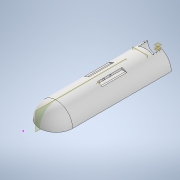
# Autodesk Inventor part: Корпус1
Saved by Autodesk Inventor 2022.1 (Build 261234000, 234)
## iProperties
Created: 2021-12-25
Part Number: Корпус1
Material: Типовые
Document SubType Name: Modeling
Designer: Grigori
Density: 1 g/cm^3
Appearance: По умолчанию
Author: Grigori
Autodesk Inventor part; units mm, degrees
ref_plane "YZ Plane" through (0, 0, 0) normal (1, 0, 0) x (0, 1, 0)
ref_plane "XZ Plane" through (0, 0, 0) normal (0, 1, 0) x (-1, 0, 0)
ref_plane "XY Plane" through (0, 0, 0) normal (0, 0, 1) x (1, 0, 0)
sketch "Эскиз1" plane through (0, 0, 0) normal (1, 0, 0) x (0, 1, 0)
  line L0 (100, -600) -> (0, -600)
  line L1 (0, -200) -> (0, -600)
  line L2 (0, -200) -> (0, -100)
  line L3 (100, -600) -> (100, -200)
  line L4 (100, -600) -> (500, -600) construction
  arc A0 (100, -200) -> (0, -100) centre (0, -200) ccw
  point P0 (0, 0)
  dimension "d0" = 100
  dimension "d4" = 100
  dimension "d42" = 400
  dimension "d43" = 90
  constraints: 10 end point, 3 vertical, 2 point on circle, 1 centre point, 1 coincident, 1 horizontal, 1 perpendicular
  measures "d0" distance of L0.start L0.end
  measures "d4" distance of L1.start L2.end
  measures "d42" distance of L3.end L0.start
  measures "d43" angle of L4 L3
extrude "Выдавливание1" add sketch "Эскиз1" along normal mid plane 500
sketch "Эскиз2" plane through (250, 100, -600) normal (0, 0, -1) x (-1, 0, 0)
  line L0 (500, -100) -> (0, -100) projected
  line L1 (-15.1415, -100) -> (-15.1415, 76.1146)
  line L2 (-15.1415, 76.1146) -> (561.5466, 76.1146)
  line L3 (561.5466, 76.1146) -> (561.5466, -100)
  line L4 (-15.1415, -100) -> (100, -100)
  line L5 (400, -100) -> (561.5466, -100)
  arc A0 (350, -100) -> (150, -100) centre (250, -100) ccw
  line L6 (100, -100) -> (150, -100)
  line L7 (350, -100) -> (400, -100)
  point P0 (150, -100)
  dimension "d44" = 200
  constraints: 14 end point, 2 collinear, 2 horizontal, 2 perpendicular, 2 point on circle, 1 centre point, 1 point on line, 1 vertical
  measures "d44" diameter of A0
extrude "Выдавливание5" cut sketch "Эскиз2" against normal through all contours L0 A0 L4 L1 L2 L3 L5
ref_plane "РабПлоскость6" through (0, 0, -600) normal (-1, 0, 0) x (0, -1, 0)
sketch "Эскиз9" plane through (0, 0, -600) normal (-1, 0, 0) x (0, -1, 0)
  arc A0 (0, 500) -> (-100, 400) centre (0, 400) ccw
  arc A1 (0, 591.5896) -> (-191.5896, 400) centre (0, 400) ccw
  line L0 (0, 400) -> (-247.1417, 400)
  line L1 (0, 400) -> (0, 629.865)
  line L2 (0, 500) -> (0, 0) projected
  point P0 (0, 600)
  constraints: 5 end point, 4 point on circle, 3 point on line, 2 centre point, 1 coincident, 1 collinear, 1 horizontal
revolve "Вращение3" cut sketch "Эскиз9" angle 360 about axis through (0, 0, -200) along (0, 0, 1) contours A0 L0 A1 L1
shell "Оболочка2" thickness 5 removed faces 1 at (33.3333, 0, -466.6667)
sketch "Эскиз11" plane through (-100, 0, -600) normal (0, -1, 0) x (1, 0, 0)
  line L0 (195, 400) -> (195, 5) projected
  line L1 (195, 5) -> (175, 5)
  line L2 (175, 5) -> (175, 25)
  line L3 (175, 25) -> (195, 25)
  line L4 (195, 25) -> (195, 5)
  line L5 (195, 5) -> (5, 5) projected
  line L6 (5, 5) -> (25, 5)
  line L7 (25, 5) -> (25, 25)
  line L8 (25, 25) -> (5, 25)
  line L9 (5, 25) -> (5, 5)
  line L10 (175, 385) -> (195, 385)
  line L11 (195, 385) -> (195, 365)
  line L12 (195, 365) -> (175, 365)
  line L13 (175, 365) -> (175, 385)
  line L14 (25, 385) -> (5, 385)
  line L15 (5, 385) -> (5, 365)
  line L16 (5, 365) -> (25, 365)
  line L17 (25, 365) -> (25, 385)
  point P0 (100, 600)
  dimension "d50" = 20
  dimension "d51" = 20
  dimension "d52" = 20
  dimension "d53" = 20
  dimension "d54" = 360
  dimension "d55" = 360
  dimension "d56" = 20
  dimension "d57" = 20
  dimension "d58" = 20
  dimension "d59" = 20
  constraints: 32 end point, 8 parallel, 4 horizontal, 4 perpendicular
  measures "d50" distance of L2.end L3.end
  measures "d51" distance of L1.end L2.end
  measures "d52" distance of L8.end L7.end
  measures "d53" distance of L7.end L6.end
  measures "d54" distance of L7.end L14.start
  measures "d55" distance of L2.end L10.start
  measures "d56" distance of L11.end L12.end
  measures "d57" distance of L10.end L11.end
  measures "d58" distance of L16.end L15.end
  measures "d59" distance of L15.end L14.end
extrude "Выдавливание6" add sketch "Эскиз11" against normal through all
sketch "Эскиз12" plane through (-100, 0, -600) normal (0, -1, 0) x (1, 0, 0)
  line L0 (195, 25) -> (175, 25) projected
  line L1 (175, 25) -> (175, 5) projected
  line L2 (25, 5) -> (25, 25) projected
  line L3 (25, 25) -> (5, 25) projected
  line L4 (5, 365) -> (25, 365) projected
  line L5 (25, 365) -> (25, 385) projected
  line L6 (175, 385) -> (175, 365) projected
  line L7 (175, 365) -> (195, 365) projected
  circle A0 centre (185, 375) radius 5
  circle A1 centre (185, 15) radius 5
  circle A2 centre (15, 15) radius 5
  circle A3 centre (15, 375) radius 5
  point P0 (100, 600)
  dimension "d62" = 10
  dimension "d63" = 10
  dimension "d64" = 10
  dimension "d65" = 10
  constraints: 4 centre point
  measures "d62" diameter of A0
  measures "d63" diameter of A1
  measures "d64" diameter of A2
  measures "d65" diameter of A3
extrude "Выдавливание7" cut sketch "Эскиз12" against normal blind 35
thread "Резьба1" size "M10x1.5" class "6H" standard "ANSI Metric M Profile" full length
thread "Резьба2" size "M10x1.5" class "6H" standard "ANSI Metric M Profile" full length
thread "Резьба3" size "M10x1.5" class "6H" standard "ANSI Metric M Profile" full length
thread "Резьба4" size "M10x1.5" class "6H" standard "ANSI Metric M Profile" full length
move faces "Перенос1" translate (0, 0, -200) faces at (-22.7518, 24.3612, -600)
shell "Оболочка3" thickness 5 removed faces 1 at (-25, 0, -731.6667)
sketch "Эскиз15" plane through (0, 0, -795) normal (0, 0, 1) x (1, 0, 0)
  arc A0 (95, 0) -> (-95, 0) centre (0, 0) ccw projected
  line L0 (95, 0) -> (-95, 0) projected
  line L1 (-95, 0) -> (95, 0)
  point P0 (0, 0)
  constraints: 2 end point, 1 horizontal
extrude "Выдавливание8" cut sketch "Эскиз15" along normal blind 201.5
sketch "Эскиз16" plane through (0, 0, -200) normal (0, -1, 0) x (1, 0, 0)
  line L0 (75, -375) -> (95, -375) projected
  line L1 (75, -393.5) -> (75, -375) projected
  line L2 (95, -375) -> (75, -375)
  line L3 (75, -375) -> (75, -393.5)
  line L4 (75, -393.5) -> (95, -393.5)
  line L5 (95, -393.5) -> (95, -375)
  line L6 (-95, -375) -> (-75, -375) projected
  line L7 (-75, -393.5) -> (-75, -375) projected
  line L8 (-95, -375) -> (-75, -375)
  line L9 (-75, -375) -> (-75, -393.5)
  line L10 (-75, -393.5) -> (-95, -393.5)
  line L11 (-95, -393.5) -> (-95, -375)
  point P0 (0, 200)
  constraints: 16 end point, 4 parallel, 2 horizontal, 2 perpendicular
extrude "Выдавливание9" add sketch "Эскиз16" against normal through all
sketch "Эскиз17" plane through (0, 0, -200) normal (0, -1, 0) x (1, 0, 0)
  line L0 (95, -375) -> (75, -375) projected
  line L1 (75, -375) -> (75, -393.5) projected
  line L2 (-75, -393.5) -> (-75, -375) projected
  line L3 (-75, -375) -> (-95, -375) projected
  circle A0 centre (-85, -384.25) radius 5
  circle A1 centre (85, -384.25) radius 5
  point P0 (0, 200)
  dimension "d84" = 10
  dimension "d85" = 10
  constraints: 2 centre point
  measures "d84" diameter of A0
  measures "d85" diameter of A1
extrude "Выдавливание10" cut sketch "Эскиз17" against normal blind 35
thread "Резьба5" size "M10x1.5" class "6H" standard "ANSI Metric M Profile" full length
thread "Резьба6" size "M10x1.5" class "6H" standard "ANSI Metric M Profile" full length
sketch "Эскиз18" plane through (0, 0, -200) normal (0, -1, 0) x (1, 0, 0)
  line L0 (-95, -595) -> (95, -595) projected
  line L1 (95, -595) -> (75, -595)
  line L2 (75, -595) -> (75, -575)
  line L3 (75, -575) -> (95, -575)
  line L4 (95, -575) -> (95, -595)
  line L5 (-95, -595) -> (-75, -595)
  line L6 (-75, -595) -> (-75, -575)
  line L7 (-75, -575) -> (-95, -575)
  line L8 (-95, -575) -> (-95, -595)
  point P0 (0, 200)
  dimension "d92" = 20
  dimension "d93" = 20
  dimension "d94" = 20
  dimension "d95" = 20
  constraints: 16 end point, 4 parallel, 2 horizontal, 2 perpendicular
  measures "d92" distance of L2.end L3.end
  measures "d93" distance of L1.end L2.end
  measures "d94" distance of L7.end L6.end
  measures "d95" distance of L6.end L5.end
extrude "Выдавливание11" add sketch "Эскиз18" against normal through all
sketch "Эскиз19" plane through (0, 0, -200) normal (0, -1, 0) x (1, 0, 0)
  line L0 (95, -575) -> (75, -575) projected
  line L1 (75, -575) -> (75, -595) projected
  line L2 (-75, -595) -> (-75, -575) projected
  line L3 (-75, -575) -> (-95, -575) projected
  circle A0 centre (-85, -585) radius 5
  circle A1 centre (85, -585) radius 5
  point P0 (0, 200)
  dimension "d98" = 10
  dimension "d99" = 10
  constraints: 2 centre point
  measures "d98" diameter of A0
  measures "d99" diameter of A1
extrude "Выдавливание12" cut sketch "Эскиз19" against normal blind 35
thread "Резьба7" size "M10x1.5" class "6H" standard "ANSI Metric M Profile" full length
thread "Резьба8" size "M10x1.5" class "6H" standard "ANSI Metric M Profile" full length
sketch "Эскиз20" plane through (0, 0, -800) normal (0, 0, -1) x (-1, 0, 0)
  line L0 (0, 0) -> (37.5, 0)
  line L1 (95, 0) -> (-95, 0) projected
  line L2 (0, 0) -> (-37.5, 0)
  line L3 (-37.5, 0) -> (-37.5, 37)
  line L4 (-37.5, 37) -> (37.5, 37)
  line L5 (37.5, 37) -> (37.5, 0)
  dimension "d106" = 37.5
  dimension "d107" = 37.5
  dimension "d108" = 37
  constraints: 10 end point, 3 perpendicular, 2 point on line
  measures "d106" distance of L0.start L0.end
  measures "d107" distance of L0.start L2.end
  measures "d108" distance of L2.end L3.end
extrude "Выдавливание13" cut sketch "Эскиз20" against normal blind 5
sketch "Эскиз21" plane through (0, 0, -800) normal (0, 0, -1) x (-1, 0, 0)
  line L0 (37.5, 37) -> (-37.5, 37) projected
  circle A0 centre (0, 84.7) radius 42.7
  point P0 (0, 0)
  constraints: 1 centre point
extrude "Выдавливание14" cut sketch "Эскиз21" against normal blind 57.7
ref_plane "РабПлоскость8" through (18.75, 37, -800) normal (0, 1, 0) x (-1, 0, 0)
sketch "Эскиз22" plane through (18.75, 37, -800) normal (0, 1, 0) x (-1, 0, 0)
  point P0 (18.75, 800)
sketch "Эскиз23" plane through (37.5, 37, -800) normal (0, 0, -1) x (-1, 0, 0)
  arc A0 (-4.7878, 53.6187) -> (79.7878, 53.6187) centre (37.5, 47.7) ccw projected
  arc A1 (-10.0891, 50.9504) -> (85.0891, 50.9504) centre (37.5, 47.7) ccw
  arc A2 (-4.7878, 53.6187) -> (-62.5, -37) centre (37.5, -37) ccw projected
  arc A3 (137.5, -37) -> (79.7878, 53.6187) centre (37.5, -37) ccw projected
  point P0 (37.5, -37)
  constraints: 2 point on circle, 1 centre point, 1 coincident
extrude "Выдавливание15" add sketch "Эскиз23" against normal blind 57.7
ref_plane "РабПлоскость10" through (18.75, 37, -800) normal (0, 1, 0) x (-1, 0, 0)
sketch "Эскиз24" plane through (18.75, 37, -800) normal (0, 1, 0) x (-1, 0, 0)
  line L0 (18.75, 97.7) -> (-1.25, 97.7)
  line L1 (18.75, 97.7) -> (38.75, 97.7)
  line L2 (38.75, 97.7) -> (38.75, 57.7)
  line L3 (-1.25, 97.7) -> (-1.25, 57.7)
  line L4 (-1.25, 57.7) -> (38.75, 57.7)
  line L5 (-23.9497, 57.7) -> (61.4497, 57.7) projected
  point P0 (18.75, 800)
  dimension "d119" = 20
  dimension "d120" = 20
  constraints: 10 end point, 2 horizontal, 1 collinear, 1 perpendicular
  measures "d119" distance of L0.start L0.end
  measures "d120" distance of L0.start L1.end
extrude "Выдавливание16" add sketch "Эскиз24" along normal through all
sketch "Эскиз25" plane through (0, 0, -742.3) normal (0, 0, -1) x (-1, 0, 0)
  line L0 (-20, 46.9735) -> (-20, 92.8709) projected
  arc A0 (-42.2878, 90.6187) -> (42.2878, 90.6187) centre (0, 84.7) ccw projected
  arc A1 (42.6997, 84.863) -> (-42.6997, 84.863) centre (0, 0) ccw projected
  line L1 (20, 46.9735) -> (20, 92.8709) projected
  arc A2 (42.6997, 84.863) -> (-42.6997, 84.863) centre (0, 0) ccw projected
  point P0 (0, 0)
extrude "Выдавливание17" add sketch "Эскиз25" against normal blind 5 contours A0 A1 L0 | L1 A1 A0
sketch "Эскиз26" plane through (18.75, 37, -800) normal (0, -1, 0) x (1, 0, 0)
  line L0 (-38.75, 97.7) -> (1.25, 97.7) projected
  line L1 (-38.75, 57.7) -> (-38.75, 97.7) projected
  line L2 (-18.75, 57.7) -> (-38.75, 57.7) projected
  line L3 (1.25, 57.7) -> (-18.75, 57.7) projected
  line L4 (1.25, 97.7) -> (1.25, 57.7) projected
  point P0 (-18.75, 800)
extrude "Выдавливание18" cut sketch "Эскиз26" against normal blind 5
ref_plane "РабПлоскость11" through (0, 0, -710.2) normal (0, 0, -1) x (-1, 0, 0)
sketch "Эскиз28" plane through (0, 0, -710.2) normal (0, 0, -1) x (-1, 0, 0)
  circle A0 centre (0, 84.7) radius 3
  point P0 (0, 0)
  constraints: 1 centre point, 1 coincident
sketch "Эскиз29" plane through (0, 0, -742.3) normal (0, 0, -1) x (-1, 0, 0)
  circle A0 centre (0, 84.7) radius 14.8
  point P0 (0, 0)
  constraints: 1 centre point, 1 coincident
loft "Лофт1" cut profiles "Эскиз28", "Эскиз29"
sketch "Эскиз31" plane through (37.5, 37, -800) normal (0, 0, -1) x (-1, 0, 0)
  circle A0 centre (-7.686, 36.724) radius 1.5
  circle A1 centre (8.1068, 11.6682) radius 1.5
  circle A2 centre (82.686, 36.724) radius 1.5
  circle A3 centre (66.8932, 11.6682) radius 1.5
  point P0 (37.5, -37)
  point P1 (85.2, 10.2)
  dimension "d140" = 3
  dimension "d141" = 3
  constraints: 4 centre point
  measures "d140" diameter of A0
  measures "d141" diameter of A1
extrude "Выдавливание19" cut sketch "Эскиз31" against normal blind 4
thread "Резьба9" size "M3x0.5" class "6H" standard "ANSI Metric M Profile" full length
thread "Резьба10" size "M3x0.5" class "6H" standard "ANSI Metric M Profile" full length
thread "Резьба11" size "M3x0.5" class "6H" standard "ANSI Metric M Profile" full length
thread "Резьба12" size "M3x0.5" class "6H" standard "ANSI Metric M Profile" full length
ref_plane "РабПлоскость12" through (18.75, 77, -800) normal (0, 1, 0) x (-1, 0, 0)
sketch "Эскиз32" plane through (18.75, 77, -800) normal (0, 1, 0) x (-1, 0, 0)
  circle A0 centre (64.6563, 52.7357) radius 1.5
  circle A1 centre (64.6563, 33.933) radius 1.5
  circle A2 centre (64.6563, 16.1937) radius 1.5
  circle A3 centre (-27.1563, 52.7357) radius 1.5
  circle A4 centre (-27.1563, 33.933) radius 1.5
  circle A5 centre (-27.1563, 16.1937) radius 1.5
  line L0 (-29.6563, 55.2357) -> (-24.6563, 55.2357)
  line L1 (-24.6563, 55.2357) -> (-24.6563, 50.2357)
  line L2 (-24.6563, 50.2357) -> (-29.6563, 50.2357)
  line L3 (-29.6563, 50.2357) -> (-29.6563, 55.2357)
  line L4 (-29.6563, 55.2357) -> (-24.6563, 50.2357) construction
  line L5 (-24.6563, 55.2357) -> (-29.6563, 50.2357) construction
  line L6 (-29.6563, 36.433) -> (-24.6563, 36.433)
  line L7 (-24.6563, 36.433) -> (-24.6563, 31.433)
  line L8 (-24.6563, 31.433) -> (-29.6563, 31.433)
  line L9 (-29.6563, 31.433) -> (-29.6563, 36.433)
  line L10 (-29.6563, 36.433) -> (-24.6563, 31.433) construction
  line L11 (-24.6563, 36.433) -> (-29.6563, 31.433) construction
  line L12 (-29.6563, 18.6937) -> (-24.6563, 18.6937)
  line L13 (-24.6563, 18.6937) -> (-24.6563, 13.6937)
  line L14 (-24.6563, 13.6937) -> (-29.6563, 13.6937)
  line L15 (-29.6563, 13.6937) -> (-29.6563, 18.6937)
  line L16 (-29.6563, 18.6937) -> (-24.6563, 13.6937) construction
  line L17 (-24.6563, 18.6937) -> (-29.6563, 13.6937) construction
  line L18 (62.1563, 18.6937) -> (67.1563, 18.6937)
  line L19 (67.1563, 18.6937) -> (67.1563, 13.6937)
  line L20 (67.1563, 13.6937) -> (62.1563, 13.6937)
  line L21 (62.1563, 13.6937) -> (62.1563, 18.6937)
  line L22 (62.1563, 18.6937) -> (67.1563, 13.6937) construction
  line L23 (67.1563, 18.6937) -> (62.1563, 13.6937) construction
  line L24 (62.1563, 36.433) -> (67.1563, 36.433)
  line L25 (67.1563, 36.433) -> (67.1563, 31.433)
  line L26 (67.1563, 31.433) -> (62.1563, 31.433)
  line L27 (62.1563, 31.433) -> (62.1563, 36.433)
  line L28 (62.1563, 36.433) -> (67.1563, 31.433) construction
  line L29 (67.1563, 36.433) -> (62.1563, 31.433) construction
  line L30 (62.1563, 55.2357) -> (67.1563, 55.2357)
  line L31 (67.1563, 55.2357) -> (67.1563, 50.2357)
  line L32 (67.1563, 50.2357) -> (62.1563, 50.2357)
  line L33 (62.1563, 50.2357) -> (62.1563, 55.2357)
  line L34 (62.1563, 55.2357) -> (67.1563, 50.2357) construction
  line L35 (67.1563, 55.2357) -> (62.1563, 50.2357) construction
  point P0 (18.75, 800)
  dimension "d159" = 3
  dimension "d160" = 3
  dimension "d161" = 3
  dimension "d162" = 5
  dimension "d163" = 5
  dimension "d164" = 5
  dimension "d165" = 5
  dimension "d166" = 5
  dimension "d167" = 5
  dimension "d168" = 5
  dimension "d169" = 5
  dimension "d170" = 5
  dimension "d171" = 5
  dimension "d172" = 5
  dimension "d173" = 5
  constraints: 72 end point, 12 midpoint, 12 parallel, 6 centre point, 6 horizontal, 6 perpendicular
  measures "d159" diameter of A0
  measures "d160" diameter of A1
  measures "d161" diameter of A2
  measures "d162" distance of L1.end L2.end
  measures "d163" distance of L0.end L1.end
  measures "d164" distance of L7.end L8.end
  measures "d165" distance of L6.end L7.end
  measures "d166" distance of L13.end L14.end
  measures "d167" distance of L12.end L13.end
  measures "d168" distance of L19.end L20.end
  measures "d169" distance of L18.end L19.end
  measures "d170" distance of L25.end L26.end
  measures "d171" distance of L24.end L25.end
  measures "d172" distance of L31.end L32.end
  measures "d173" distance of L30.end L31.end
extrude "Выдавливание20" add sketch "Эскиз32" along normal blind 4 and the other way blind 12 contours A3 | A4 | A5 | L0 L1 L2 L3 | L6 L7 L8 L9 | L12 L13 L14 L15 | L18 L19 L20 L21 | L24 L25 L26 L27 | L30 L31 L32 L33
sketch "Эскиз33" plane through (18.75, 65, -800) normal (0, -1, 0) x (1, 0, 0)
  circle A0 centre (-64.6563, 52.7357) radius 1.5 projected
  circle A1 centre (-64.6563, 33.933) radius 1.5 projected
  circle A2 centre (-64.6563, 16.1937) radius 1.5 projected
  line L0 (18.75, 0) -> (-56.25, 0) projected
  line L1 (-18.75, 0) -> (-18.75, 65.1849)
  circle A3 centre (27.1563, 52.7357) radius 1.5
  circle A4 centre (27.1563, 33.933) radius 1.5
  circle A5 centre (27.1563, 16.1937) radius 1.5
  line L2 (-18.75, 0) -> (27.1563, 0)
  line L3 (18.75, 0) -> (81.25, 0) projected
  point P0 (-18.75, 800)
  point P1 (-67.1563, 50.2357)
  point P2 (-62.1919, 50.2357)
  constraints: 4 end point, 3 centre point, 3 symmetric about line, 1 midpoint, 1 point on line, 1 vertical, 3 other
extrude "Выдавливание21" cut sketch "Эскиз33" against normal through all
ref_plane "РабПлоскость13" through (18.75, 100.5, -800) normal (0, 1, 0) x (-1, 0, 0)
sketch "Эскиз34" plane through (18.75, 100.5, -800) normal (0, 1, 0) x (-1, 0, 0)
  line L0 (-81.25, 0) -> (-81.25, 600) projected
  line L1 (18.75, 375) -> (48.75, 375)
  line L2 (48.75, 375) -> (48.75, 225)
  line L3 (48.75, 225) -> (18.75, 225)
  line L4 (18.75, 225) -> (-11.25, 225)
  line L5 (-11.25, 225) -> (-11.25, 375)
  line L6 (-11.25, 375) -> (18.75, 375)
  line L7 (48.75, 375) -> (78.75, 375)
  line L8 (78.75, 375) -> (78.75, 225)
  line L9 (78.75, 225) -> (48.75, 225)
  line L10 (48.75, 225) -> (48.75, 375)
  line L11 (-11.25, 375) -> (-41.25, 375)
  line L12 (-41.25, 375) -> (-41.25, 225)
  line L13 (-41.25, 225) -> (-11.25, 225)
  line L14 (-11.25, 225) -> (-11.25, 375)
  point P0 (18.75, 800)
  point P1 (-11.25, 225)
  dimension "d236" = 30
  dimension "d238" = 30
  dimension "d239" = 30
  constraints: 28 end point, 6 parallel, 4 horizontal, 4 perpendicular, 2 point on line
  measures "d236" distance of L2.end L3.end
  measures "d238" distance of L8.end L9.end
  measures "d239" distance of L13.end L12.end
ref_plane "РабПлоскость17" through (18.75, 84.063, -800) normal (0, 1, 0) x (1, 0, 0)
extrude "Выдавливание29" cut sketch "Эскиз34" against normal blind 16.437 contours L7 L8 L9 L2 | L5 L13 L12 L11
sketch "Эскиз47" plane through (18.75, 37, -800) normal (0, 1, 0) x (-1, 0, 0)
  line L0 (-11.25, 375) -> (-11.25, 225) projected
  line L1 (-11.25, 375) -> (48.75, 375)
  line L2 (-11.25, 225) -> (48.75, 225)
  line L3 (-25.5039, 375) -> (-25.5039, 225) projected
  line L4 (63.0039, 225) -> (63.0039, 375) projected
  line L5 (48.75, 375) -> (63.0039, 375) projected
  line L6 (-25.5039, 375) -> (-11.25, 375) projected
  line L7 (-11.25, 225) -> (-25.5039, 225) projected
  line L8 (63.0039, 225) -> (48.75, 225) projected
  point P0 (18.75, 800)
  constraints: 4 end point, 1 parallel, 1 perpendicular
extrude "Выдавливание31" add sketch "Эскиз47" along normal blind 58.5
sketch "Эскиз50" plane through (18.75, 37, -800) normal (0, -1, 0) x (1, 0, 0)
  line L0 (25.5039, 225) -> (-63.0039, 225) projected
  line L1 (-63.0039, 375) -> (25.5039, 375) projected
  line L2 (-72.911, 225) -> (-63.0039, 225) projected
  line L3 (-63.0039, 225) -> (-63.0039, 223)
  line L4 (-63.0039, 225) -> (-61.0039, 225) construction
  line L5 (-63.0039, 223) -> (25.5039, 223)
  line L6 (25.5039, 225) -> (35.411, 225) projected
  line L7 (25.5039, 223) -> (25.5039, 225)
  line L8 (-63.0039, 375) -> (-63.0039, 377)
  line L9 (-63.0039, 375) -> (-61.0039, 375) construction
  line L10 (-63.0039, 377) -> (25.5039, 377)
  line L11 (25.5039, 377) -> (25.5039, 375)
  point P0 (-18.75, 800)
  dimension "d251" = 2
  dimension "d252" = 90
  dimension "d253" = 2
  dimension "d254" = 90
  constraints: 16 end point, 6 perpendicular, 2 horizontal, 2 vertical
  measures "d251" distance of L0.end L3.end
  measures "d252" angle of L3 L4
  measures "d253" distance of L1.start L8.end
  measures "d254" angle of L9 L8
extrude "Выдавливание33" add sketch "Эскиз50" against normal through all
sketch "Эскиз51" plane through (18.75, 37, -800) normal (0, -1, 0) x (1, 0, 0)
  line L0 (-63.0039, 377) -> (-63.0039, 223) projected
  line L1 (-63.0039, 223) -> (25.5039, 223) projected
  line L2 (25.5039, 223) -> (25.5039, 377) projected
  line L3 (25.5039, 377) -> (-63.0039, 377) projected
  point P0 (-18.75, 800)
extrude "Выдавливание34" cut sketch "Эскиз51" against normal blind 43
ref_plane "РабПлоскость20" through (30, 84.063, -425) normal (1, 0, 0) x (0, 0, -1)
sketch "Эскиз53" plane through (18.75, 100.5, -800) normal (0, 1, 0) x (-1, 0, 0)
  line L0 (-11.25, 375) -> (18.75, 375)
  line L1 (-11.25, 375) -> (-41.25, 375)
  line L2 (18.75, 375) -> (48.75, 375)
  line L3 (48.75, 375) -> (78.75, 375)
  line L4 (-41.25, 375) -> (-41.25, 225)
  line L5 (78.75, 375) -> (78.75, 225)
  line L6 (18.75, 225) -> (-11.25, 225)
  line L7 (-41.25, 225) -> (-11.25, 225)
  line L8 (48.75, 225) -> (18.75, 225)
  line L9 (78.75, 225) -> (48.75, 225)
  line L10 (-25.5039, 225) -> (63.0039, 225)
  line L11 (48.75, 375) -> (43.75, 375)
  line L12 (43.75, 375) -> (43.75, 225)
  line L13 (43.75, 225) -> (48.75, 225)
  line L14 (-25.5039, 375) -> (63.0039, 375)
  line L15 (-11.25, 225) -> (-6.25, 225)
  line L16 (-6.25, 225) -> (-6.25, 375)
  line L17 (-6.25, 375) -> (-11.25, 375)
  point P0 (18.75, 800)
  point P1 (-6.25, 225)
  point P2 (-6.25, 375)
  dimension "d262" = 30
  dimension "d263" = 30
  dimension "d264" = 30
  dimension "d265" = 5
  dimension "d266" = 5
  constraints: 36 end point, 6 horizontal, 6 parallel, 4 perpendicular, 4 point on line
  measures "d262" distance of L8.start L8.end
  measures "d263" distance of L5.end L9.end
  measures "d264" distance of L15.start L4.end
  measures "d265" distance of L13.end L12.end
  measures "d266" distance of L17.end L17.start
extrude "Выдавливание35" cut sketch "Эскиз53" against normal blind 16.437 contours L0 L16 L6 L7 L4 L1 | L2 L3 L5 L9 L8 L12
sketch "Эскиз54" plane through (25, 84.063, -425) normal (1, 0, 0) x (0, 0, -1)
  circle A0 centre (38.5008, 6) radius 5
  circle A1 centre (78.7009, 6) radius 5
  line L0 (150, 0) -> (0, 0) projected
  line L1 (38.5008, 0) -> (44.5008, 0) construction
  point P0 (-425, -84.063)
  dimension "d269" = 10
  constraints: 2 centre point, 2 end point, 1 horizontal, 1 point on line
  measures "d269" diameter of A1
extrude "Выдавливание36" cut sketch "Эскиз54" against normal through all
